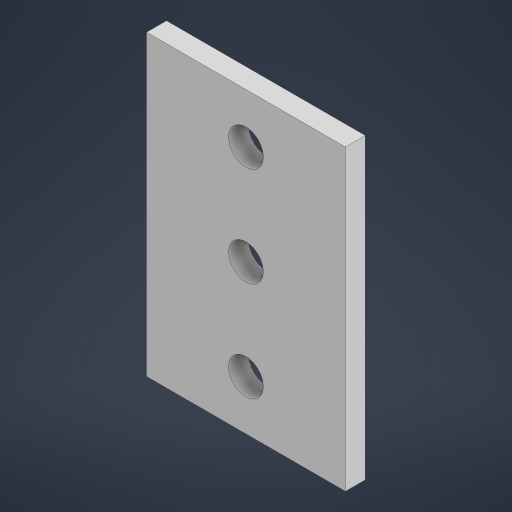
# Autodesk Inventor part: top spacer
Saved by Autodesk Inventor 2023 (Build 270158000, 158)
## iProperties
Created: 2022-06-04
Part Number: top spacer
Material: Generic
Document SubType Name: Modeling
Designer: vibhu
Density: 1 g/cm^3
Appearance: Default
Author: vibhu
Autodesk Inventor part; units mm, degrees
ref_plane "YZ Plane" through (0, 0, 0) normal (1, 0, 0) x (0, 1, 0)
ref_plane "XZ Plane" through (0, 0, 0) normal (0, 1, 0) x (-1, 0, 0)
ref_plane "Work Plane1" through (0, 0, 0) normal (0, 0, 1) x (1, 0, 0)
sketch "Sketch1" plane through (0, 0, 0) normal (0, 0, 1) x (1, 0, 0)
  circle A0 centre (10, 5) radius 1.75 projected
  circle A1 centre (10, 25) radius 1.75 projected
  circle A2 centre (10, 15) radius 1.75 projected
  line L0 (20, 30) -> (0, 30) projected
  line L1 (0, 0) -> (0, 30) projected
  line L2 (20, 0) -> (0, 0) projected
  line L3 (20, 0) -> (20, 30) projected
extrude "Extrusion1" add sketch "Sketch1" along normal blind 2
body "Solid1"
